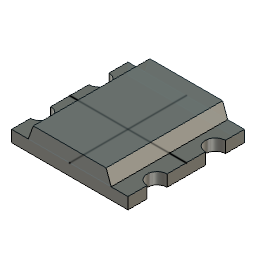
rgbled (Autodesk Fusion 360 design; units mm, degrees)
part number: 2025-12-16-13-41-37-580
Autodesk Fusion 360 part; units mm, degrees
sketch "Sketch1" plane through (0, 0, 0) normal (0, 0, 1) x (1, 0, 0)
  line L0 (0, 0) -> (1.6, 0)
  line L1 (1.6, 0) -> (1.6, 1.6)
  line L2 (1.6, 1.6) -> (0, 1.6)
  line L3 (0, 1.6) -> (0, 0)
  line L4 (0.4, 1.6) -> (0, 1.6)
  line L5 (0.4, 1.6) -> (1.2, 1.6)
  line L6 (1.2, 1.6) -> (1.2, 0)
  line L7 (1.2, 0) -> (0.4, 0)
  line L8 (0.4, 0) -> (0.4, 1.6)
  line L9 (0, 1.6) -> (0.125, 1.6)
  line L10 (0.125, 1.6) -> (1.475, 1.6)
  line L11 (1.475, 1.6) -> (1.475, 0)
  line L12 (1.475, 0) -> (0.125, 0)
  line L13 (0.125, 0) -> (0.125, 1.6)
  line L14 (1.6, 0.8) -> (0, 0.8)
  line L15 (0.8, 1.6) -> (0.8, 0)
  line L16 (0, 1.6) -> (0, 1.475)
  line L17 (0, 1.475) -> (0.275, 1.475)
  line L18 (0.275, 1.475) -> (0.275, 0.925)
  line L19 (0.275, 0.925) -> (0, 0.925)
  line L20 (0, 0.925) -> (0, 1.475)
  circle A0 centre (0, 1.2) radius 0.1375
  circle A1 centre (1.6, 1.2) radius 0.1375
  line L21 (1.6, 0.925) -> (1.6, 1.475)
  line L22 (1.6, 1.475) -> (1.325, 1.475)
  line L23 (1.325, 1.475) -> (1.325, 0.925)
  line L24 (1.325, 0.925) -> (1.6, 0.925)
  circle A2 centre (1.6, 0.4) radius 0.1375
  line L25 (1.6, 1.6) -> (1.6, 0)
  line L26 (1.6, 0.125) -> (1.325, 0.125)
  line L27 (1.325, 0.125) -> (1.325, 0.675)
  line L28 (1.325, 0.675) -> (1.6, 0.675)
  circle A3 centre (0, 0.4) radius 0.1375
  line L29 (0, 1.6) -> (0, 0)
  line L30 (0.275, 0.675) -> (0, 0.675)
  line L31 (0.275, 0.125) -> (0.275, 0.675)
  line L32 (0, 0.125) -> (0.275, 0.125)
  dimension "d1" = 1.6
  dimension "d2" = 1.6
  dimension "d3" = 0.8
  dimension "d4" = 1.6
  dimension "d5" = 0.125
  dimension "d6" = 1.35
  dimension "d7" = 1.6
  dimension "d8" = 0.125
  dimension "d9" = 0.275
  dimension "d10" = 0.55
  dimension "d11" = 0.275
  constraint horizontal L0
  constraint vertical L1
  constraint horizontal L2
  constraint vertical L3
  constraint coincident L0.start L3.end
  constraint coincident L2 L4.start
  constraint horizontal L5
  constraint vertical L6
  constraint horizontal L7
  constraint vertical L8
  constraint coincident L2 L9.end
  constraint horizontal L10
  constraint vertical L11
  constraint horizontal L12
  constraint vertical L13
  constraint midpoint L1 L14.start
  constraint midpoint L3 L14.end
  constraint midpoint L10 L15.start
  constraint midpoint L0 L15.end
  constraint perpendicular L9 L16
  constraint horizontal L17
  constraint vertical L18
  constraint horizontal L19
  constraint vertical L20
  constraint midpoint L20 A0.centre
  constraint symmetric L15 L16.end L21.end
  constraint symmetric L15 L17.end L22.end
  constraint symmetric L15 L18.end L23.end
  constraint symmetric L15 L19.end L21.start
  constraint symmetric L15 A0 A1
  constraint symmetric L0.end L14 L1.end
  constraint symmetric L1.end L14 L0.end
  constraint symmetric L14 A1 A2
  constraint symmetric L14 L21.start L28.end
  constraint symmetric L14 L21.end L26.start
  constraint symmetric L14 L22.end L26.end
  constraint symmetric L14 L23.end L27.end
  constraint symmetric L15 A2 A3
  constraint symmetric L15 L1.end L2.end
  constraint symmetric L15 L0.end L0.start
  constraint symmetric L15 L26.start L32.start
  constraint symmetric L15 L26.end L31.start
  constraint symmetric L15 L27.end L30.start
  constraint symmetric L15 L28.end L30.end
  measures "d1" distance of L0.start L0.end
  measures "d2" distance of L0.start L2.end
  measures "d3" distance of L4.start L5.end
  measures "d4" distance of L4.start L7.end
  measures "d5" distance of L2.end L9.end
  measures "d6" distance of L9.end L10.end
  measures "d7" distance of L9.end L12.end
  measures "d8" distance of L2.end L16.end
  measures "d9" distance of L16.end L17.end
  measures "d10" distance of L16.end L19.end
  measures "d11" diameter of A0
extrude "Extrude1" add sketch "Sketch1" along normal blind 0.16 contours L0 L3 L13 L29 L32 | L0 L8 L12 L13 L14 L30 L31 L32 | L3 L13 A3 L29 L32 | L0 L7 L8 L12 L14 L15 | L13 A3 L30 L31 L32 | L0 L6 L7 L12 L14 L15 | L2 L4 L8 L10 L13 L14 L17 L18 L19 | L2 L5 L8 L10 L14 L15 | L3 L13 A3 L29 L30 | L0 L6 L11 L12 L14 L26 L27 L28 | L2 L5 L6 L10 L14 L15 | L3 L13 L14 L19 L29 | L3 L13 L14 L29 L30 | L0 L1 L11 L25 L26 | L2 L6 L10 L11 L14 L22 L23 L24 | L2 L3 L4 L9 L13 L16 L17 L29 | L3 L13 L19 L20 A0 L29 | L13 L17 L18 L19 A0 | L11 A2 L26 L27 L28 | L1 L11 A2 L25 L26 | L1 L11 L14 L25 L28 | L1 L11 L14 L24 L25 | L3 L13 L17 L20 A0 L29 | L1 L2 L11 L22 L25 | L11 A1 L22 L23 L24 | L1 L11 A1 L21 L24 L25 | L1 L11 A2 L25 L28 | L1 L11 A1 L21 L22 L25
sketch "Sketch2" plane through (0, 0, 0.16) normal (0, 0, 1) x (-1, 0, 0)
  line L0 (-1.6, -1.6) -> (0, -1.6)
  line L1 (0, -1.6) -> (0, -1.3375)
  arc A0 (0, -1.0625) -> (0, -1.3375) centre (0, -1.2) ccw
  line L2 (0, -1.0625) -> (0, -0.5375)
  arc A1 (0, -0.2625) -> (0, -0.5375) centre (0, -0.4) ccw
  line L3 (0, -0.2625) -> (0, 0)
  line L4 (0, 0) -> (-1.6, 0)
  line L5 (-1.6, 0) -> (-1.6, -0.2625)
  arc A2 (-1.6, -0.5375) -> (-1.6, -0.2625) centre (-1.6, -0.4) ccw
  line L6 (-1.6, -0.5375) -> (-1.6, -1.0625)
  arc A3 (-1.6, -1.3375) -> (-1.6, -1.0625) centre (-1.6, -1.2) ccw
  line L7 (-1.6, -1.3375) -> (-1.6, -1.6)
  line L8 (-0.8, -1.6) -> (-0.8, 0)
  line L9 (0, -0.8) -> (-1.6, -0.8)
  constraint midpoint L0 L8.start
  constraint midpoint L4 L8.end
  constraint midpoint L2 L9.start
  constraint midpoint L6 L9.end
sketch "Sketch3" plane through (0, 0, 0.16) normal (0, 0, 1) x (-1, 0, 0)
  line L0 (0, -1.6) -> (-0.25, -1.6)
  line L1 (-0.25, -1.6) -> (-1.35, -1.6)
  line L2 (-1.35, -1.6) -> (-1.35, 0)
  line L3 (-1.35, 0) -> (-0.25, 0)
  line L4 (-0.25, 0) -> (-0.25, -1.6)
  dimension "d14" = 0.25
  dimension "d15" = 1.1
  dimension "d16" = 1.6
  constraint horizontal L0
  constraint horizontal L1
  constraint vertical L2
  constraint horizontal L3
  constraint vertical L4
  measures "d14" distance of L0.start L0.end
  measures "d15" distance of L0.end L1.end
  measures "d16" distance of L0.end L3.end
extrude "Extrude2" add sketch "Sketch3" along normal blind 0.19
sketch "Sketch4" plane through (0, 0, 0.35) normal (0, 0, 1) x (-1, 0, 0)
  line L0 (-0.25, 0) -> (-1.35, 0)
  line L1 (-1.35, 0) -> (-1.35, -1.6)
  line L2 (-1.35, -1.6) -> (-0.25, -1.6)
  line L3 (-0.25, -1.6) -> (-0.25, 0)
  line L4 (-1.35, 0) -> (-1.3, 0)
  line L5 (-1.3, 0) -> (-1.3, -1.6)
  line L6 (-1.3, -1.6) -> (-1.35, -1.6)
  line L7 (-1.35, -1.6) -> (-1.35, 0)
  line L8 (-0.8, 0) -> (-0.8, -1.6)
  line L9 (-0.25, -1.6) -> (-0.25, 0)
  line L10 (-0.3, 0) -> (-0.3, -1.6)
  dimension "d19" = 0.05
  constraint horizontal L4
  constraint vertical L5
  constraint horizontal L6
  constraint vertical L7
  constraint coincident L0.end L1.start
  constraint midpoint L0 L8.start
  constraint midpoint L2 L8.end
  constraint symmetric L0.end L8 L0.start
  constraint symmetric L4.end L8 L10.start
  constraint symmetric L5.end L8 L10.end
  constraint symmetric L1.end L8 L2.end
  measures "d19" distance of L0.end L4.end
extrude "Extrude3" cut sketch "Sketch4" against normal blind 0.19 contours L0 L2 L3 L9 L10 | L0 L1 L2 L4 L5 L6 L7
sketch "Sketch5" plane through (0, 0, 0.35) normal (0, 0, 1) x (-1, 0, 0)
  line L0 (-0.3, -1.6) -> (-0.3, 0)
  line L1 (-0.3, 0) -> (-1.3, 0)
  line L2 (-1.3, 0) -> (-1.3, -1.6)
  line L3 (-1.3, -1.6) -> (-0.3, -1.6)
draft "Draft1" angle 20 neutral plane through (0, 0, 0.35) pull (0, 0, 1) 1 faces at (1.3, 0.5333, 0.2867)
draft "Draft2" angle 20 neutral plane through (0, 0, 0.35) pull (0, 0, 1) 1 faces at (0.3, 0.5333, 0.2867)
sketch "Sketch6" plane through (0, 1.6, 0) normal (0, 1, 0) x (-1, 0, 0)
  line L0 (-0.2308, 0.16) -> (-0.3, 0.35)
  line L1 (-0.3, 0.35) -> (-1.3, 0.35)
  line L2 (-1.3, 0.35) -> (-1.3692, 0.16)
  line L3 (-1.3692, 0.16) -> (-1.6, 0.16)
  line L4 (-1.6, 0.16) -> (-1.6, 0)
  line L5 (-1.6, 0) -> (0, 0)
  line L6 (0, 0) -> (0, 0.16)
  line L7 (0, 0.16) -> (-0.2308, 0.16)
